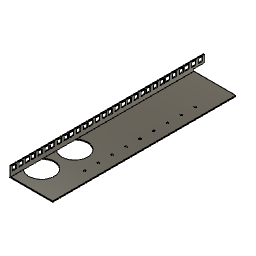
TV Cabinet Rack Posts (Autodesk Fusion 360 design; units mm, degrees)
Autodesk Fusion 360 part; units mm, degrees
sketch "Sketch1" plane through (0, 0, 0) normal (0, 0, 1) x (1, 0, 0) in component "Rack Posts"
  line L0 (-75, 326) -> (24, 326)
  line L1 (24, 326) -> (24, -98)
  line L2 (24, -98) -> (-75, -98)
  line L3 (-75, -98) -> (-75, 326)
  circle A0 centre (0, 0) radius 2.5
  circle A1 centre (0, 32) radius 2.5
  circle A2 centre (0, 64) radius 2.5
  circle A3 centre (0, 96) radius 2.5
  circle A4 centre (0, 128) radius 2.5
  circle A5 centre (0, 160) radius 2.5
  circle A6 centre (0, 192) radius 2.5
  circle A7 centre (0, 224) radius 2.5
  circle A8 centre (0, 256) radius 2.5
  circle A9 centre (-54, 31) radius 30
  line L4 (0, 1.75) -> (0, 22.5)
  line L5 (1.75, 0) -> (22.5, 0)
  circle A10 centre (-54, -46) radius 30
  dimension "d1195" = 75
  dimension "d1196" = 24
  dimension "d1197" = 98
  dimension "d1198" = 326
  dimension "d1199" = 5
  dimension "d1202" = 0
  dimension "d1203" = 32
  dimension "d1204" = 60
  dimension "d1205" = 54
  dimension "d1206" = 31
  dimension "d1209" = 0
  dimension "d1210" = -77
  constraint horizontal L0
  constraint vertical L1
  constraint horizontal L2
  constraint vertical L3
  constraint coincident A0.centre origin
  measures "d1195" distance of A0.centre L3
  measures "d1196" distance of A0.centre L1
  measures "d1197" distance of A0.centre L2
  measures "d1198" distance of A0.centre L0
  measures "d1199" diameter of A0
  measures "d1204" diameter of A9
  measures "d1205" distance of A9.centre L4
  measures "d1206" distance of A9.centre L5
extrude "Extrude3" add sketch "Sketch1" along normal blind 1.981 contours L0 L1 L2 L3 A9 A10 in component "Rack Posts"
sketch "Sketch4" plane through (-75, 0, 0) normal (-1, 0, 0) x (0, -1, 0) in component "Rack Posts"
  line L0 (67.4243, 0) -> (98, 0)
  line L1 (98, 0) -> (98, 1.981)
  line L2 (98, 1.981) -> (67.4243, 1.981)
  line L3 (67.4243, 1.981) -> (67.4243, 0)
  line L4 (98, 1.981) -> (-326, 1.981)
  line L5 (-326, 1.981) -> (-326, 24)
  line L6 (-326, 24) -> (98, 24)
  line L7 (98, 24) -> (98, 1.981)
  line L8 (98, 0) -> (-326, 0)
  line L9 (-326, 4) -> (-326, 24)
  line L10 (-346.5, 21.75) -> (-337, 21.75)
  line L11 (-337, 21.75) -> (-337, 12.25)
  line L12 (-337, 12.25) -> (-346.5, 12.25)
  line L13 (-346.5, 12.25) -> (-346.5, 21.75)
  line L14 (-330.625, 21.75) -> (-321.125, 21.75)
  line L15 (-321.125, 21.75) -> (-321.125, 12.25)
  line L16 (-321.125, 12.25) -> (-330.625, 12.25)
  line L17 (-330.625, 12.25) -> (-330.625, 21.75)
  line L18 (-314.75, 21.75) -> (-305.25, 21.75)
  line L19 (-305.25, 21.75) -> (-305.25, 12.25)
  line L20 (-305.25, 12.25) -> (-314.75, 12.25)
  line L21 (-314.75, 12.25) -> (-314.75, 21.75)
  line L22 (-302.05, 21.75) -> (-292.55, 21.75)
  line L23 (-292.55, 21.75) -> (-292.55, 12.25)
  line L24 (-292.55, 12.25) -> (-302.05, 12.25)
  line L25 (-302.05, 12.25) -> (-302.05, 21.75)
  line L26 (-286.175, 12.25) -> (-286.175, 21.75)
  line L27 (-286.175, 21.75) -> (-276.675, 21.75)
  line L28 (-276.675, 21.75) -> (-276.675, 12.25)
  line L29 (-276.675, 12.25) -> (-286.175, 12.25)
  line L30 (-260.8, 21.75) -> (-260.8, 12.25)
  line L31 (-270.3, 21.75) -> (-260.8, 21.75)
  line L32 (-270.3, 12.25) -> (-270.3, 21.75)
  line L33 (-260.8, 12.25) -> (-270.3, 12.25)
  line L34 (-257.6, 21.75) -> (-248.1, 21.75)
  line L35 (-248.1, 21.75) -> (-248.1, 12.25)
  line L36 (-248.1, 12.25) -> (-257.6, 12.25)
  line L37 (-257.6, 12.25) -> (-257.6, 21.75)
  line L38 (-241.725, 12.25) -> (-241.725, 21.75)
  line L39 (-241.725, 21.75) -> (-232.225, 21.75)
  line L40 (-232.225, 21.75) -> (-232.225, 12.25)
  line L41 (-232.225, 12.25) -> (-241.725, 12.25)
  line L42 (-216.35, 21.75) -> (-216.35, 12.25)
  line L43 (-225.85, 21.75) -> (-216.35, 21.75)
  line L44 (-225.85, 12.25) -> (-225.85, 21.75)
  line L45 (-216.35, 12.25) -> (-225.85, 12.25)
  line L46 (-213.15, 21.75) -> (-203.65, 21.75)
  line L47 (-203.65, 21.75) -> (-203.65, 12.25)
  line L48 (-203.65, 12.25) -> (-213.15, 12.25)
  line L49 (-213.15, 12.25) -> (-213.15, 21.75)
  line L50 (-197.275, 12.25) -> (-197.275, 21.75)
  line L51 (-197.275, 21.75) -> (-187.775, 21.75)
  line L52 (-187.775, 21.75) -> (-187.775, 12.25)
  line L53 (-187.775, 12.25) -> (-197.275, 12.25)
  line L54 (-171.9, 21.75) -> (-171.9, 12.25)
  line L55 (-181.4, 21.75) -> (-171.9, 21.75)
  line L56 (-181.4, 12.25) -> (-181.4, 21.75)
  line L57 (-171.9, 12.25) -> (-181.4, 12.25)
  line L58 (-168.7, 21.75) -> (-159.2, 21.75)
  line L59 (-159.2, 21.75) -> (-159.2, 12.25)
  line L60 (-159.2, 12.25) -> (-168.7, 12.25)
  line L61 (-168.7, 12.25) -> (-168.7, 21.75)
  line L62 (-152.825, 12.25) -> (-152.825, 21.75)
  line L63 (-152.825, 21.75) -> (-143.325, 21.75)
  line L64 (-143.325, 21.75) -> (-143.325, 12.25)
  line L65 (-143.325, 12.25) -> (-152.825, 12.25)
  line L66 (-127.45, 21.75) -> (-127.45, 12.25)
  line L67 (-136.95, 21.75) -> (-127.45, 21.75)
  line L68 (-136.95, 12.25) -> (-136.95, 21.75)
  line L69 (-127.45, 12.25) -> (-136.95, 12.25)
  line L70 (-124.25, 21.75) -> (-114.75, 21.75)
  line L71 (-114.75, 21.75) -> (-114.75, 12.25)
  line L72 (-114.75, 12.25) -> (-124.25, 12.25)
  line L73 (-124.25, 12.25) -> (-124.25, 21.75)
  line L74 (-108.375, 12.25) -> (-108.375, 21.75)
  line L75 (-108.375, 21.75) -> (-98.875, 21.75)
  line L76 (-98.875, 21.75) -> (-98.875, 12.25)
  line L77 (-98.875, 12.25) -> (-108.375, 12.25)
  line L78 (-83, 21.75) -> (-83, 12.25)
  line L79 (-92.5, 21.75) -> (-83, 21.75)
  line L80 (-92.5, 12.25) -> (-92.5, 21.75)
  line L81 (-83, 12.25) -> (-92.5, 12.25)
  line L82 (-79.8, 21.75) -> (-70.3, 21.75)
  line L83 (-70.3, 21.75) -> (-70.3, 12.25)
  line L84 (-70.3, 12.25) -> (-79.8, 12.25)
  line L85 (-79.8, 12.25) -> (-79.8, 21.75)
  line L86 (-63.925, 12.25) -> (-63.925, 21.75)
  line L87 (-63.925, 21.75) -> (-54.425, 21.75)
  line L88 (-54.425, 21.75) -> (-54.425, 12.25)
  line L89 (-54.425, 12.25) -> (-63.925, 12.25)
  line L90 (-38.55, 21.75) -> (-38.55, 12.25)
  line L91 (-48.05, 21.75) -> (-38.55, 21.75)
  line L92 (-48.05, 12.25) -> (-48.05, 21.75)
  line L93 (-38.55, 12.25) -> (-48.05, 12.25)
  line L94 (-35.35, 21.75) -> (-25.85, 21.75)
  line L95 (-25.85, 21.75) -> (-25.85, 12.25)
  line L96 (-25.85, 12.25) -> (-35.35, 12.25)
  line L97 (-35.35, 12.25) -> (-35.35, 21.75)
  line L98 (-19.475, 12.25) -> (-19.475, 21.75)
  line L99 (-19.475, 21.75) -> (-9.975, 21.75)
  line L100 (-9.975, 21.75) -> (-9.975, 12.25)
  line L101 (-9.975, 12.25) -> (-19.475, 12.25)
  line L102 (5.9, 21.75) -> (5.9, 12.25)
  line L103 (-3.6, 21.75) -> (5.9, 21.75)
  line L104 (-3.6, 12.25) -> (-3.6, 21.75)
  line L105 (5.9, 12.25) -> (-3.6, 12.25)
  line L106 (9.1, 21.75) -> (18.6, 21.75)
  line L107 (18.6, 21.75) -> (18.6, 12.25)
  line L108 (18.6, 12.25) -> (9.1, 12.25)
  line L109 (9.1, 12.25) -> (9.1, 21.75)
  line L110 (24.975, 12.25) -> (24.975, 21.75)
  line L111 (24.975, 21.75) -> (34.475, 21.75)
  line L112 (34.475, 21.75) -> (34.475, 12.25)
  line L113 (34.475, 12.25) -> (24.975, 12.25)
  line L114 (50.35, 21.75) -> (50.35, 12.25)
  line L115 (40.85, 21.75) -> (50.35, 21.75)
  line L116 (40.85, 12.25) -> (40.85, 21.75)
  line L117 (50.35, 12.25) -> (40.85, 12.25)
  line L118 (53.55, 21.75) -> (63.05, 21.75)
  line L119 (63.05, 21.75) -> (63.05, 12.25)
  line L120 (63.05, 12.25) -> (53.55, 12.25)
  line L121 (53.55, 12.25) -> (53.55, 21.75)
  line L122 (69.425, 12.25) -> (69.425, 21.75)
  line L123 (69.425, 21.75) -> (78.925, 21.75)
  line L124 (78.925, 21.75) -> (78.925, 12.25)
  line L125 (78.925, 12.25) -> (69.425, 12.25)
  line L126 (94.8, 21.75) -> (94.8, 12.25)
  line L127 (85.3, 21.75) -> (94.8, 21.75)
  line L128 (85.3, 12.25) -> (85.3, 21.75)
  line L129 (94.8, 12.25) -> (85.3, 12.25)
  line L130 (-326, 24) -> (-349.7, 24)
  line L131 (-349.7, 24) -> (-349.7, 7)
  line L132 (-349.7, 7) -> (-326, 7)
  line L133 (-326, 7) -> (-326, 24)
  point P0 (-326, 1.981)
  point P1 (-326, 0)
  dimension "d1254" = 9.5
  dimension "d1255" = 9.5
  dimension "d1260" = 15.875
  dimension "d1261" = 0
  dimension "d1264" = 44.45
  dimension "d1265" = 0
  dimension "d1268" = 7
  dimension "d1269" = 447.7
  dimension "d1270" = 24
  constraint horizontal L4
  constraint vertical L5
  constraint horizontal L6
  constraint vertical L7
  constraint coincident L1.end L2.start
  constraint coincident L5 P0
  constraint vertical L9
  constraint horizontal L10
  constraint vertical L11
  constraint horizontal L12
  constraint vertical L13
  constraint horizontal L130
  constraint vertical L131
  constraint horizontal L132
  constraint vertical L133
  measures "d1254" distance of L10.start L10.end
  measures "d1255" distance of L10.start L12.end
  measures "d1268" distance of P1 L132
  measures "d1269" distance of L7 L131
  measures "d1270" distance of L6 L8
extrude "Extrude6" add sketch "Sketch4" against normal blind 1.981 contours L2 L4 L5 L6 L7 L9 L14 L15 L16 L133 | L5 L9 L14 L16 L17 L130 L131 L132 L133 in component "Rack Posts"
component "Rack Posts" placed x (1, 0, 0) y (0, 1, 0) z (0, 0, 1) at (0, 0, 0)
